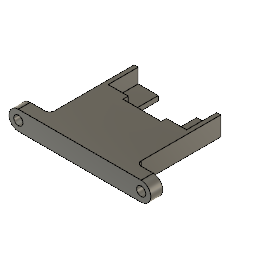
LED_Matrix_Halterung (Autodesk Fusion 360 design; units mm, degrees)
Autodesk Fusion 360 part; units mm, degrees
sketch "Skizze1" plane through (0, 0, 0) normal (0, 0, 1) x (1, 0, 0)
  line L0 (0, 0) -> (36, 0)
  line L1 (36, 0) -> (36, -8)
  line L2 (36, -8) -> (0, -8)
  line L3 (0, -8) -> (0, 0)
  line L4 (24, 0) -> (24, -3)
  line L5 (24, -3) -> (12, -3)
  line L6 (12, -3) -> (12, 0)
  dimension "d1" = 36
  dimension "d2" = 8
  dimension "d3" = 12
  dimension "d4" = 3
  dimension "d5" = 12
  measures "d2" distance of L0.start
  measures "d3" distance of L0.start
  measures "d5" distance of L3 L6
extrude "Extrusion1" add sketch "Skizze1" along normal blind 40 contours L0 L1 L2 L3 L4 L5 L6
sketch "Skizze3" plane through (0, 0, 40) normal (0, 0, 1) x (-1, 0, 0)
  line L0 (-24, 0) -> (-24, 3)
  line L1 (-24, 3) -> (-12, 3)
  line L2 (-12, 3) -> (-12, 0)
  line L3 (-12, 0) -> (0, 0)
  line L4 (0, 0) -> (0, 8)
  line L5 (0, 8) -> (-36, 8)
  line L6 (-36, 8) -> (-36, 0)
  line L7 (-36, 0) -> (-24, 0)
  line L8 (-1.75, 2) -> (-34.25, 2)
  line L9 (-34.25, 2) -> (-34.25, 8)
  line L10 (-34.25, 8) -> (-1.75, 8)
  line L11 (-1.75, 8) -> (-1.75, 2)
extrude "Extrusion3" cut sketch "Skizze3" against normal blind 12 contours L0 L1 L2 L5 L8 L9 L10 L11
sketch "Skizze4" plane through (0, 0, 0) normal (0, 0, 1) x (1, 0, 0)
  line L0 (12, 0) -> (24, 0)
  line L1 (24, 0) -> (24, -3)
  line L2 (24, -3) -> (12, -3)
  line L3 (12, -3) -> (12, 0)
extrude "Extrusion4" add sketch "Skizze4" along normal blind 26.5
sketch "Skizze5" plane through (0, 0, 0) normal (0, 0, 1) x (1, 0, 0)
  line L0 (0, -8) -> (0, 0)
  line L1 (0, 0) -> (0, -8)
  line L2 (0, -4) -> (-12, -4)
  line L3 (0, 0) -> (-8, 0)
  line L4 (0, -8) -> (-8, -8)
  arc A0 (-8, 0) -> (-8, -8) centre (-8, -4) ccw
  line L5 (36, -8) -> (0, -8)
  line L6 (17.4652, 5.0702) -> (17.4652, -10)
  arc A1 (42.9304, -8) -> (42.9304, 0) centre (42.9304, -4) ccw
  line L7 (34.9304, 0) -> (42.9304, 0)
  line L8 (34.9304, -8) -> (42.9304, -8)
  line L9 (34.9304, 0) -> (34.9304, -8)
  dimension "d15" = 12
  dimension "d28" = 8
  dimension "d29" = 8
  dimension "d30" = 8
  measures "d29" distance of L0.end
  measures "d30" distance of L3 L4
extrude "Extrusion5" add sketch "Skizze5" along normal blind 5
fillet "Abrundung2" radius 2 2 edges at (36, -4, 5) (0, -4, 5)
sketch "Skizze6" plane through (0, 0, 5) normal (0, 0, 1) x (-1, 0, 0)
  line L0 (-38, 0) -> (-38, 8)
  line L1 (-38, 8) -> (-42.9304, 8)
  arc A0 (-42.9304, 8) -> (-42.9304, 0) centre (-42.9304, 4) ccw
  line L2 (-42.9304, 0) -> (-38, 0)
  circle A1 centre (-42.9304, 4) radius 1.9
  circle A2 centre (8, 4) radius 1.9
  line L3 (0, 0) -> (0, 8)
  dimension "d19" = 3.8
  dimension "d20" = 3.8
  dimension "d31" = 8
  measures "d19" diameter of A1
  measures "d20" diameter of A2
  measures "d31" distance of L3
extrude "Extrusion6" cut sketch "Skizze6" against normal blind 5 contours A1 | A2
move_body "Verschieben2" bodies 1 to x (1, 0, 0) y (0, 0, -1) z (0, 1, 0) at (0, 0, 0)
sketch "Skizze8" plane through (0, 28, 0) normal (0, 1, 0) x (-1, 0, 0)
  line L0 (-24, 2) -> (-24, 3)
  line L1 (-12, 3) -> (-12, 2)
  line L2 (-12, 2) -> (-1.75, 2)
  line L3 (-1.75, 2) -> (-1.75, 8)
  line L4 (-1.75, 8) -> (-34.25, 8)
  line L5 (-34.25, 8) -> (-34.25, 2)
  line L6 (-34.25, 2) -> (-24, 2)
  line L7 (-24, 3) -> (-12, 3)
  line L8 (-12, 3) -> (-12, 8)
  line L9 (-12, 8) -> (-24, 8)
  line L10 (-24, 8) -> (-24, 3)
  line L11 (-24, 3) -> (-12, 3)
extrude "Extrusion8" add sketch "Skizze8" against normal blind 3 contours L4 L7 L8 L9 L10 L11
sketch "Skizze9" plane through (0, 28, 0) normal (0, 1, 0) x (-1, 0, 0)
  line L0 (-1.75, 8) -> (-34.25, 8)
  line L1 (-34.25, 8) -> (-34.25, 2)
  line L2 (-34.25, 2) -> (-24, 2)
  line L3 (-24, 2) -> (-24, 3)
  line L4 (-12, 3) -> (-12, 2)
  line L5 (-12, 2) -> (-1.75, 2)
  line L6 (-1.75, 2) -> (-1.75, 8)
  line L7 (-24, 3) -> (-12, 3)
  line L8 (-12, 3) -> (-12, 8)
  line L9 (-12, 8) -> (-24, 8)
  line L10 (-24, 8) -> (-24, 3)
  line L11 (-24, 3) -> (-12, 3)
extrude "Extrusion9" cut sketch "Skizze9" against normal blind 1.5 contours L0 L7 L8 L9 L10 L11
move_face "Flächen versetzen1" offset -0.4 2 faces at (12, 27, 4.6667) (12, 31.5, 0.6667)
move_face "Flächen versetzen2" offset -0.4 1 faces at (24, 31.5, 0.6667)
move_face "Flächen versetzen3" offset -1.5 1 faces at (24.4, 31.5, 0.6667)
move_face "Flächen versetzen4" offset -1.5 2 faces at (11.6, 27.5, 4.6667) (11.6, 31.5, 0.6667)
move_face "Flächen versetzen5" offset -0.2 1 faces at (20.6333, 26.5, 3.6667)
move_face "Flächen versetzen6" offset -1 1 faces at (20.6333, 26.3, 3.6667)
move_face "Flächen versetzen7" offset -0.5 1 faces at (4.5333, 28, 4.3333)
move_face "Flächen versetzen8" offset -0.5 1 faces at (31.4667, 28, 6)
